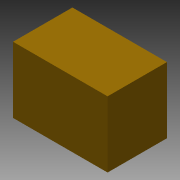
# Autodesk Inventor part: CX2156NL
Saved by Autodesk Inventor 2015 SP1 (Build 190203100, 203)
## iProperties
Created: 2015-10-19
Part Number: CX2156NL
Material: Generic
Document SubType Name: Modeling
Designer: Kartikye
Density: 1 g/cm^3
Appearance: CX2156NL, CX2156NL
Author: Kartikye
Autodesk Inventor part; units mm, degrees
ref_plane "YZ Plane" through (0, 0, 0) normal (1, 0, 0) x (0, 1, 0)
ref_plane "XZ Plane" through (0, 0, 0) normal (0, 1, 0) x (-1, 0, 0)
ref_plane "XY Plane" through (0, 0, 0) normal (0, 0, 1) x (1, 0, 0)
sketch "CX2156NL, CX2156NL_5" plane through (0, 0, 0) normal (0, 0, 1) x (1, 0, 0)
  line L0 (3.3, -1.7) -> (-1, -1.7)
  line L1 (-1, -1.7) -> (-1, 1)
  line L2 (-1, 1) -> (3.3, 1)
  line L3 (3.3, 1) -> (3.3, -1.7)
  dimension "d2" = 4.3
  dimension "d3" = 2.7
  constraints: 8 end point
  measures "d2" distance of L1.end L2.end
  measures "d3" distance of L0.end L1.end
extrude "Extrusion1" add sketch "CX2156NL, CX2156NL_5" along normal blind 3
body "Solid1"
